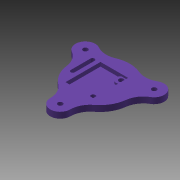
# Autodesk Inventor part: Gyro Mount
Saved by Autodesk Inventor 2014 (Build 180170000, 170)
## iProperties
Created: 2014-02-06
Part Number: Gyro Mount
Material: Generic
Document SubType Name: Modeling
Designer: Spooner
Density: 1 g/cm^3
Appearance: Violet
Mass: 5.01972 g
Surface Area: 42.8108 cm^2
Volume: 5.01972 cm^3
Author: Spooner
Autodesk Inventor part; units mm, degrees
ref_plane "YZ Plane" through (0, 0, 0) normal (1, 0, 0) x (0, 1, 0)
ref_plane "XZ Plane" through (0, 0, 0) normal (0, 1, 0) x (-1, 0, 0)
ref_plane "XY Plane" through (0, 0, 0) normal (0, 0, 1) x (1, 0, 0)
sketch "Sketch1" plane through (0, 0, 0) normal (0, 1, 0) x (-1, 0, 0)
  arc A0 (6.35, 25.4) -> (-6.35, 25.4) centre (0, 25.4) ccw
  arc A1 (-11.43, 15.24) -> (11.43, 15.24) centre (0, 0) ccw
  arc A2 (-11.43, 15.24) -> (-6.35, 25.4) centre (-19.05, 25.4) ccw
  arc A3 (6.35, 25.4) -> (11.43, 15.24) centre (19.05, 25.4) ccw
  dimension "d0" = 25.4
  dimension "d1" = 38.1
  dimension "d2" = 12.7
  constraints: 8 point on circle, 4 centre point, 4 tangent, 2 horizontal alignment, 1 coincident, 1 vertical alignment
  measures "d0" distance of A0.centre A1.centre
  measures "d1" diameter of A1
  measures "d2" diameter of A0
extrude "Extrusion1" add sketch "Sketch1" along normal blind 3.81
sketch "Sketch2" plane through (0, 3.81, 0) normal (0, 1, 0) x (1, 0, 0)
  arc A0 (-6.35, -25.4) -> (6.35, -25.4) centre (0, -25.4) ccw projected
  circle A1 centre (0, -25.4) radius 1.524
  dimension "d5" = 3.048
  constraints: 1 centre point, 1 coincident
  measures "d5" diameter of A1
extrude "Extrusion2" cut sketch "Sketch2" against normal through all
pattern_circular "Circular Pattern1" count 3 over 360 about axis through (0, 0, 0) along (0, 1, 0) of "Extrusion2", "Extrusion1"
sketch "Sketch3" plane through (0, 3.81, 0) normal (0, 1, 0) x (1, 0, 0)
  arc A0 (11.43, -15.24) -> (18.9132, -2.2787) centre (0, 0) ccw projected
  line L0 (-10.2616, 10.6299) -> (7.3914, 10.6299)
  line L1 (7.3914, 10.6299) -> (7.3914, -11.7221)
  line L2 (7.3914, -11.7221) -> (-10.2616, -11.7221)
  line L3 (-10.2616, -11.7221) -> (-10.2616, 10.6299)
  dimension "d11" = 22.352
  dimension "d12" = 17.653
  dimension "d14" = 10.6299
  dimension "d29" = 7.3914
  constraints: 8 end point, 2 parallel, 1 horizontal, 1 perpendicular
  measures "d11" distance of L2.end L0.start
  measures "d12" distance of L1.end L2.end
  measures "d14" distance from line of A0.centre L0
  measures "d29" distance from line of L1 A0.centre
extrude "Extrusion3" cut sketch "Sketch3" against normal blind 2.54
sketch "Sketch4" plane through (0, 1.27, 0) normal (0, 1, 0) x (1, 0, 0)
  line L0 (-10.2616, 10.6299) -> (7.3914, 10.6299) projected
  line L1 (7.3914, -11.7221) -> (-10.2616, -11.7221) projected
  line L2 (7.3914, 10.6299) -> (7.3914, -11.7221) projected
  circle A0 centre (5.1816, 8.4201) radius 1.524
  circle A1 centre (5.1816, -9.5123) radius 1.524
  point P0 (0, 0)
  dimension "d17" = 3.048
  dimension "d18" = 2.2098
  dimension "d19" = 2.2098
  dimension "d20" = 2.2098
  constraints: 2 centre point, 1 equal radius, 1 vertical alignment
  measures "d17" diameter of A0
  measures "d18" distance from line of L2 A0.centre
  measures "d19" distance from line of L0 A0.centre
  measures "d20" distance from line of L1 A1.centre
extrude "Extrusion4" cut sketch "Sketch4" against normal through all
sketch "Sketch5" plane through (0, 1.27, 0) normal (0, 1, 0) x (1, 0, 0)
  circle A0 centre (5.1816, 8.4201) radius 1.524 projected
  circle A1 centre (5.1816, -9.5123) radius 1.524 projected
  line L0 (-10.2616, 10.6299) -> (7.3914, 10.6299) projected
  circle A2 centre (5.1816, 8.4201) radius 3.175
  circle A3 centre (5.1816, -9.5123) radius 3.175
  point P0 (0, 0)
  dimension "d31" = 6.35
  constraints: 2 centre point, 2 coincident, 1 equal radius
  measures "d31" diameter of A2
extrude "Extrusion5" add sketch "Sketch5" along normal blind 1.27
sketch "Sketch6" plane through (0, 3.81, 0) normal (0, 1, 0) x (1, 0, 0)
  line L0 (-10.2616, -11.7221) -> (-10.2616, 10.6299) projected
  line L1 (-10.2616, 10.6299) -> (7.3914, 10.6299) projected
  line L2 (-12.8016, 9.3599) -> (-12.8016, -3.3401)
  line L3 (-15.3416, -3.3401) -> (-15.3416, 9.3599)
  arc A0 (-12.8016, 9.3599) -> (-15.3416, 9.3599) centre (-14.0716, 9.3599) ccw
  arc A1 (-15.3416, -3.3401) -> (-12.8016, -3.3401) centre (-14.0716, -3.3401) ccw
  point P0 (-12.8016, -11.7221)
  dimension "d25" = 2.54
  dimension "d26" = 2.54
  dimension "d30" = 12.7
  constraints: 5 tangent, 4 end point, 4 point on circle, 2 centre point, 1 horizontal alignment, 1 parallel
  measures "d25" distance between parallel lines of L0 L2
  measures "d26" distance between parallel lines of L2 L3
  measures "d30" distance of A0.centre A1.centre
extrude "Extrusion6" cut sketch "Sketch6" against normal through all
equation "\"d19\" = d18"
equation "\"d20\" = d18"
body "Solid1"
